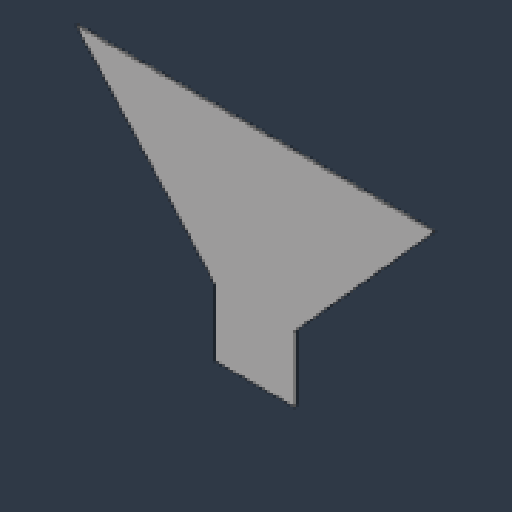
# Autodesk Inventor part: trough_backplate
Saved by Autodesk Inventor 2024.3 (Build 283343000, 343)
## iProperties
Created: 2025-03-03
Part Number: trough_backplate
Material: Generic
Document SubType Name: Sheet Metal
Designer: marcu
Density: 1 g/cm^3
Sheet Metal Rule: Default
Appearance: Default
Mass: 475.838 g
Surface Area: 3181.35 cm^2
Volume: 475.838 cm^3
Author: marcu
Autodesk Inventor part; units mm, degrees
ref_plane "YZ Plane" through (0, 0, 0) normal (1, 0, 0) x (0, 1, 0)
ref_plane "XZ Plane" through (0, 0, 0) normal (0, 1, 0) x (-1, 0, 0)
ref_plane "XY Plane" through (0, 0, 0) normal (0, 0, 1) x (1, 0, 0)
sketch "Sketch1" plane through (0, 0, 0) normal (0, 0, 1) x (1, 0, 0)
  line L0 (374.65, -215.9) -> (-374.65, -215.9)
  line L1 (-374.65, -215.9) -> (-374.65, 215.9)
  line L2 (-374.65, 215.9) -> (374.65, 215.9)
  line L3 (374.65, 215.9) -> (374.65, -215.9)
  line L4 (374.65, -215.9) -> (-374.65, 215.9) construction
  line L5 (-374.65, -215.9) -> (374.65, 215.9) construction
  line L6 (-374.65, -88.9) -> (374.65, -88.9) construction
  line L7 (-374.65, 215.9) -> (-76.2, -88.9)
  line L8 (374.65, 215.9) -> (76.2, -88.9)
  line L9 (-76.2, -88.9) -> (-76.2, -215.9)
  line L10 (76.2, -88.9) -> (76.2, -215.9)
  line L11 (-349.25, 189.9596) -> (-349.25, 215.9)
  line L12 (349.25, 215.9) -> (349.25, 189.9596)
  point P0 (0, 0)
  dimension "d0" = 749.3
  dimension "d1" = 431.8
  dimension "d5" = 152.4
  dimension "d6" = 76.2
  dimension "d7" = 127
  dimension "d8" = 25.4
  dimension "d9" = 25.4
  measures "d0" distance of L1.end L2.end
  measures "d1" distance of L0.end L1.end
  measures "d5" distance of L8.end L7.end
  measures "d6" horizontal distance of point (0, 0) L8.end
  measures "d7" distance between parallel lines of L0 L6
  measures "d8" distance between parallel lines of L1 L11
  measures "d9" distance between parallel lines of L3 L12
extrude "Plate1" add sketch "Sketch1" along normal blind 3.048 contours L0 L9 L7 L11 L2 L12 L8 L10
equation "\"d2\" = Thickness"
equation "\"BendRadius\" = Thickness"
equation "\"BendReliefWidth\" = Thickness"
equation "\"BendReliefDepth\" = 0.5 * Thickness"
equation "\"CornerReliefSize\" = 4 * Thickness"
equation "\"MinimumRemnant\" = 2 * Thickness"
equation "\"TransitionRadius\" = BendRadius"
equation "\"JacobiRadiusSize\" = BendRadius"
equation "\"GapSize\" = Thickness"
equation "\"Thickness\" = 3.048"
body "Solid1"
